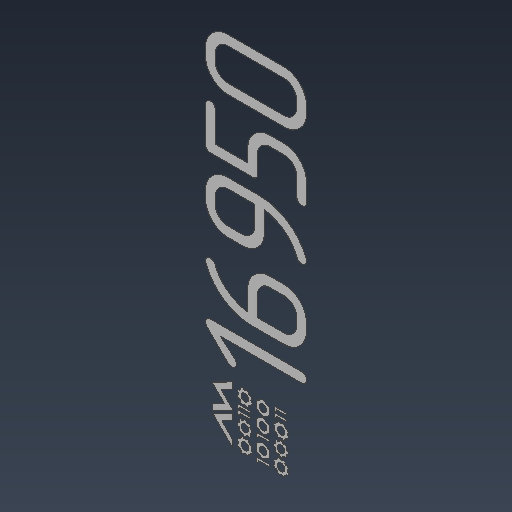
# Autodesk Inventor part: цифры
Saved by Autodesk Inventor 2025 (Build 290162000, 162)
## iProperties
Created: 2025-03-07
Part Number: цифры
Material: Типовые
Document SubType Name: Modeling
Designer: GameHD
Density: 1 g/cm^3
Appearance: По умолчанию
Author: GameHD
Autodesk Inventor part; units mm, degrees
ref_plane "YZ Plane" through (0, 0, 0) normal (1, 0, 0) x (0, 1, 0)
ref_plane "XZ Plane" through (0, 0, 0) normal (0, 1, 0) x (-1, 0, 0)
ref_plane "XY Plane" through (0, 0, 0) normal (0, 0, 1) x (1, 0, 0)
sketch "Эскиз1" plane through (0, 0, 0) normal (0, 0, 1) x (1, 0, 0)
  arc A0 (27.3071, -95.8521) -> (31.3071, -91.8521) centre (27.3071, -91.8521) ccw
  line L0 (31.3071, 96.2479) -> (31.3071, -91.8521)
  arc A1 (31.3071, 96.2479) -> (28.3071, 99.2479) centre (28.3071, 96.2479) ccw
  line L1 (-29.1929, 99.2479) -> (28.3071, 99.2479)
  arc A2 (-29.1929, 99.2479) -> (-32.1929, 96.2479) centre (-29.1929, 96.2479) ccw
  line L2 (-32.1929, -91.8521) -> (-32.1929, 96.2479)
  arc A3 (-32.1929, -91.8521) -> (-28.1929, -95.8521) centre (-28.1929, -91.8521) ccw
  line L3 (-28.1929, -95.8521) -> (27.3071, -95.8521)
  line L4 (-18.208, -66.6682) -> (-12.464, -72.4126)
  line L5 (-12.464, -72.4126) -> (-12.464, -72.9974)
  line L6 (-12.464, -72.9974) -> (-22.3101, -77.9492)
  line L7 (-22.3101, -77.9492) -> (-22.3101, -74.8598)
  line L8 (-22.3101, -74.8598) -> (-16.5747, -71.9754)
  line L9 (-16.5747, -71.9754) -> (-22.3101, -66.2395)
  line L10 (-22.3101, -66.2395) -> (-22.3101, -65.617)
  line L11 (-22.3101, -65.617) -> (-12.464, -60.6652)
  line L12 (-12.464, -60.6652) -> (-12.485, -63.79)
  line L13 (-12.485, -63.79) -> (-18.208, -66.6682)
  line L14 (-5.5283, -89.0998) -> (-5.7626, -88.5746)
  arc A4 (-6.7374, -88.5729) -> (-5.7626, -88.5746) centre (-6.2446, -85.4284) ccw
  line L15 (-6.7374, -88.5729) -> (-6.9459, -89.1173)
  arc A5 (-8.3342, -88.531) -> (-6.9459, -89.1173) centre (-6.8364, -86.9215) ccw
  line L16 (-8.3342, -88.531) -> (-8.1285, -87.9939)
  arc A6 (-8.8166, -87.3034) -> (-8.1285, -87.9939) centre (-6.2446, -85.4284) ccw
  line L17 (-8.8166, -87.3034) -> (-9.349, -87.5409)
  arc A7 (-9.916, -86.1447) -> (-9.349, -87.5409) centre (-7.7189, -86.0657) ccw
  line L18 (-9.916, -86.1447) -> (-9.3907, -85.9104)
  arc A8 (-9.3891, -84.9356) -> (-9.3907, -85.9104) centre (-6.2446, -85.4284) ccw
  line L19 (-9.3891, -84.9356) -> (-9.9335, -84.7271)
  arc A9 (-9.3471, -83.3388) -> (-9.9335, -84.7271) centre (-7.7377, -84.8366) ccw
  line L20 (-9.3471, -83.3388) -> (-8.81, -83.5445)
  arc A10 (-8.1196, -82.8564) -> (-8.81, -83.5445) centre (-6.2446, -85.4284) ccw
  line L21 (-8.1196, -82.8564) -> (-8.3571, -82.324)
  arc A11 (-6.9608, -81.757) -> (-8.3571, -82.324) centre (-6.8819, -83.9541) ccw
  line L22 (-6.9608, -81.757) -> (-6.7265, -82.2822)
  arc A12 (-5.7517, -82.2839) -> (-6.7265, -82.2822) centre (-6.2446, -85.4284) ccw
  line L23 (-5.7517, -82.2839) -> (-5.5432, -81.7395)
  arc A13 (-4.155, -82.3259) -> (-5.5432, -81.7395) centre (-5.6527, -83.9353) ccw
  line L24 (-4.155, -82.3259) -> (-4.3713, -82.8744)
  arc A14 (-3.6832, -83.5648) -> (-4.3713, -82.8744) centre (-6.2552, -85.4398) ccw
  line L25 (-3.6832, -83.5648) -> (-3.1508, -83.3273)
  arc A15 (-2.5838, -84.7236) -> (-3.1508, -83.3273) centre (-4.7809, -84.8025) ccw
  line L26 (-2.5838, -84.7236) -> (-3.109, -84.9579)
  arc A16 (-3.1107, -85.9327) -> (-3.109, -84.9579) centre (-6.2552, -85.4398) ccw
  line L27 (-3.1107, -85.9327) -> (-2.5663, -86.1412)
  arc A17 (-3.142, -87.518) -> (-2.5663, -86.1412) centre (-4.7621, -86.0318) ccw
  line L28 (-3.142, -87.518) -> (-3.6791, -87.3123)
  arc A18 (-4.3696, -88.0004) -> (-3.6791, -87.3123) centre (-6.2446, -85.4284) ccw
  line L29 (-4.3696, -88.0004) -> (-4.132, -88.5328)
  arc A19 (-5.5283, -89.0998) -> (-4.132, -88.5328) centre (-5.6073, -86.9027) ccw
  line L30 (-9.8069, -73.459) -> (-9.8069, -71.4081)
  line L31 (-9.8069, -71.4081) -> (-3.4639, -71.4081)
  line L32 (-3.4639, -71.4081) -> (-3.4639, -72.491)
  line L33 (-3.4639, -72.491) -> (-8.6953, -72.491)
  line L34 (-8.6953, -72.491) -> (-8.6953, -73.459)
  line L35 (-8.6953, -73.459) -> (-9.8069, -73.459)
  line L36 (-0.4429, -89.1671) -> (-0.4429, -87.1162)
  line L37 (-0.4429, -87.1162) -> (5.9001, -87.1162)
  line L38 (5.9001, -87.1162) -> (5.9001, -88.1992)
  line L39 (5.9001, -88.1992) -> (0.6687, -88.1992)
  line L40 (0.6687, -88.1992) -> (0.6687, -89.1671)
  line L41 (0.6687, -89.1671) -> (-0.4429, -89.1671)
  line L42 (8.3427, -65.5184) -> (8.3427, -63.4675)
  line L43 (8.3427, -63.4675) -> (14.6857, -63.4675)
  line L44 (14.6857, -63.4675) -> (14.6857, -64.5504)
  line L45 (14.6857, -64.5504) -> (9.4543, -64.5504)
  line L46 (9.4543, -64.5504) -> (9.4543, -65.5184)
  line L47 (9.4543, -65.5184) -> (8.3427, -65.5184)
  arc A20 (11.322, -88.5729) -> (12.2968, -88.5746) centre (11.8148, -85.4284) ccw
  line L48 (11.322, -88.5729) -> (11.1135, -89.1173)
  arc A21 (9.7252, -88.531) -> (11.1135, -89.1173) centre (11.223, -86.9215) ccw
  line L49 (9.7252, -88.531) -> (9.9309, -87.9939)
  arc A22 (9.2428, -87.3034) -> (9.9309, -87.9939) centre (11.8148, -85.4284) ccw
  line L50 (9.2428, -87.3034) -> (8.7104, -87.5409)
  arc A23 (8.1434, -86.1447) -> (8.7104, -87.5409) centre (10.3405, -86.0657) ccw
  line L51 (8.1434, -86.1447) -> (8.6686, -85.9104)
  arc A24 (8.6703, -84.9356) -> (8.6686, -85.9104) centre (11.8148, -85.4284) ccw
  line L52 (8.6703, -84.9356) -> (8.1259, -84.7271)
  arc A25 (8.7123, -83.3388) -> (8.1259, -84.7271) centre (10.3217, -84.8366) ccw
  line L53 (8.7123, -83.3388) -> (9.2493, -83.5445)
  arc A26 (9.9398, -82.8564) -> (9.2493, -83.5445) centre (11.8148, -85.4284) ccw
  line L54 (9.9398, -82.8564) -> (9.7023, -82.324)
  arc A27 (11.0986, -81.757) -> (9.7023, -82.324) centre (11.1775, -83.9541) ccw
  line L55 (11.0986, -81.757) -> (11.3329, -82.2822)
  arc A28 (12.3077, -82.2839) -> (11.3329, -82.2822) centre (11.8148, -85.4284) ccw
  line L56 (12.3077, -82.2839) -> (12.5162, -81.7395)
  arc A29 (13.9044, -82.3259) -> (12.5162, -81.7395) centre (12.4067, -83.9353) ccw
  line L57 (13.9044, -82.3259) -> (13.6987, -82.8629)
  arc A30 (14.3868, -83.5534) -> (13.6987, -82.8629) centre (11.8148, -85.4284) ccw
  line L58 (14.3868, -83.5534) -> (14.9192, -83.3159)
  arc A31 (15.4862, -84.7122) -> (14.9192, -83.3159) centre (13.2891, -84.7911) ccw
  line L59 (15.4862, -84.7122) -> (14.961, -84.9465)
  arc A32 (14.9593, -85.9213) -> (14.961, -84.9465) centre (11.8148, -85.4284) ccw
  line L60 (14.9593, -85.9213) -> (15.5037, -86.1298)
  arc A33 (14.9174, -87.518) -> (15.5037, -86.1298) centre (13.3079, -86.0203) ccw
  line L61 (14.9174, -87.518) -> (14.3803, -87.3123)
  arc A34 (13.6898, -88.0004) -> (14.3803, -87.3123) centre (11.8148, -85.4284) ccw
  line L62 (13.6898, -88.0004) -> (13.9273, -88.5328)
  arc A35 (12.5311, -89.0998) -> (13.9273, -88.5328) centre (12.4521, -86.9027) ccw
  line L63 (12.5311, -89.0998) -> (12.2968, -88.5746)
  line L64 (8.3427, -62.7161) -> (8.3427, -60.6652)
  line L65 (8.3427, -60.6652) -> (14.6857, -60.6652)
  line L66 (14.6857, -60.6652) -> (14.6857, -61.7481)
  line L67 (14.6857, -61.7481) -> (9.4543, -61.7481)
  line L68 (9.4543, -61.7481) -> (9.4543, -62.7161)
  line L69 (9.4543, -62.7161) -> (8.3427, -62.7161)
  line L70 (-0.4429, -78.55) -> (-0.4429, -76.4991)
  line L71 (-0.4429, -76.4991) -> (5.9001, -76.4991)
  line L72 (5.9001, -76.4991) -> (5.9001, -77.5821)
  line L73 (5.9001, -77.5821) -> (0.6687, -77.5821)
  line L74 (0.6687, -77.5821) -> (0.6687, -78.55)
  line L75 (0.6687, -78.55) -> (-0.4429, -78.55)
  line L76 (-3.4639, -69.8464) -> (-8.6953, -69.8464)
  line L77 (-8.6953, -69.8464) -> (-8.6953, -70.8144)
  line L78 (-8.6953, -70.8144) -> (-9.8069, -70.8144)
  line L79 (-9.8069, -70.8144) -> (-9.8069, -68.7635)
  line L80 (-9.8069, -68.7635) -> (-3.4639, -68.7635)
  line L81 (-3.4639, -68.7635) -> (-3.4639, -69.8464)
  line L82 (-22.3101, -79.2695) -> (-12.464, -74.2847)
  line L83 (-12.464, -74.2847) -> (-12.464, -77.3998)
  line L84 (-12.464, -77.3998) -> (-17.7048, -80.0531)
  line L85 (-17.7048, -80.0531) -> (-12.464, -85.531)
  line L86 (-12.464, -85.531) -> (-12.464, -89.0892)
  line L87 (-12.464, -89.0892) -> (-22.3101, -79.2695)
  arc A36 (-7.8758, -80.1695) -> (-7.029, -80.513) centre (-6.3219, -77.554) ccw
  line L88 (-7.8758, -80.1695) -> (-8.3322, -80.5742)
  arc A37 (-9.3244, -79.5396) -> (-8.3322, -80.5742) centre (-7.1141, -78.4131) ccw
  line L89 (-9.3244, -79.5396) -> (-8.9143, -79.1463)
  arc A38 (-9.2702, -78.3047) -> (-8.9143, -79.1463) centre (-6.3219, -77.554) ccw
  line L90 (-9.2702, -78.3047) -> (-9.8791, -78.2681)
  arc A39 (-9.849, -76.8349) -> (-9.8791, -78.2681) centre (-7.4896, -77.6013) ccw
  line L91 (-9.849, -76.8349) -> (-9.2809, -76.8468)
  arc A40 (-8.9375, -76.0001) -> (-9.2809, -76.8468) centre (-6.3219, -77.554) ccw
  line L92 (-8.9375, -76.0001) -> (-9.3422, -75.5437)
  arc A41 (-8.3075, -74.5515) -> (-9.3422, -75.5437) centre (-7.1811, -76.7617) ccw
  line L93 (-8.3075, -74.5515) -> (-7.9143, -74.9616)
  arc A42 (-7.0727, -74.6057) -> (-7.9143, -74.9616) centre (-6.3219, -77.554) ccw
  line L94 (-7.0727, -74.6057) -> (-7.0361, -73.9968)
  arc A43 (-5.6029, -74.0268) -> (-7.0361, -73.9968) centre (-6.3693, -76.3863) ccw
  line L95 (-5.6029, -74.0268) -> (-5.6148, -74.5949)
  arc A44 (-4.7681, -74.9384) -> (-5.6148, -74.5949) centre (-6.3219, -77.554) ccw
  line L96 (-4.7681, -74.9384) -> (-4.3116, -74.5337)
  arc A45 (-3.3195, -75.5683) -> (-4.3116, -74.5337) centre (-5.5297, -76.6948) ccw
  line L97 (-3.3195, -75.5683) -> (-3.7296, -75.9616)
  arc A46 (-3.3737, -76.8032) -> (-3.7296, -75.9616) centre (-6.3219, -77.554) ccw
  line L98 (-3.3737, -76.8032) -> (-2.7648, -76.8398)
  arc A47 (-2.7948, -78.273) -> (-2.7648, -76.8398) centre (-5.1542, -77.5066) ccw
  line L99 (-2.7948, -78.273) -> (-3.3629, -78.2611)
  arc A48 (-3.7063, -79.1078) -> (-3.3629, -78.2611) centre (-6.3219, -77.554) ccw
  line L100 (-3.7063, -79.1078) -> (-3.3016, -79.5642)
  arc A49 (-4.3363, -80.5564) -> (-3.3016, -79.5642) centre (-5.4628, -78.3462) ccw
  line L101 (-4.3363, -80.5564) -> (-4.7296, -80.1463)
  arc A50 (-5.5712, -80.5022) -> (-4.7296, -80.1463) centre (-6.3219, -77.554) ccw
  line L102 (-5.5712, -80.5022) -> (-5.6078, -81.1111)
  arc A51 (-7.0409, -81.0811) -> (-5.6078, -81.1111) centre (-6.2746, -78.7216) ccw
  line L103 (-7.0409, -81.0811) -> (-7.029, -80.513)
  line L104 (5.9001, -80.9599) -> (5.9001, -84.6242)
  line L105 (5.9001, -84.6242) -> (2.6904, -86.4378)
  line L106 (2.6904, -86.4378) -> (-0.4429, -84.6242)
  line L107 (-0.4429, -84.6242) -> (-0.4429, -80.9599)
  line L108 (-0.4429, -80.9599) -> (2.7668, -79.1463)
  line L109 (2.7668, -79.1463) -> (5.9001, -80.9599)
  line L110 (2.7668, -60.7467) -> (5.9001, -62.5603)
  line L111 (5.9001, -62.5603) -> (5.9001, -66.2246)
  line L112 (5.9001, -66.2246) -> (2.6904, -68.0382)
  line L113 (2.6904, -68.0382) -> (-0.4429, -66.2246)
  line L114 (-0.4429, -66.2246) -> (-0.4429, -62.5603)
  line L115 (-0.4429, -62.5603) -> (2.7668, -60.7467)
  arc A52 (12.4882, -80.5022) -> (13.3298, -80.1463) centre (11.7375, -77.554) ccw
  line L116 (12.4882, -80.5022) -> (12.4516, -81.1111)
  arc A53 (11.0184, -81.0811) -> (12.4516, -81.1111) centre (11.7848, -78.7216) ccw
  line L117 (11.0184, -81.0811) -> (11.0303, -80.513)
  arc A54 (10.1836, -80.1695) -> (11.0303, -80.513) centre (11.7375, -77.554) ccw
  line L118 (10.1836, -80.1695) -> (9.7272, -80.5742)
  arc A55 (8.735, -79.5396) -> (9.7272, -80.5742) centre (10.9453, -78.4131) ccw
  line L119 (8.735, -79.5396) -> (9.1451, -79.1463)
  arc A56 (8.7892, -78.3047) -> (9.1451, -79.1463) centre (11.7375, -77.554) ccw
  line L120 (8.7892, -78.3047) -> (8.1803, -78.2681)
  arc A57 (8.2104, -76.8349) -> (8.1803, -78.2681) centre (10.5698, -77.6013) ccw
  line L121 (8.2104, -76.8349) -> (8.7784, -76.8468)
  arc A58 (9.1219, -76.0001) -> (8.7784, -76.8468) centre (11.7375, -77.554) ccw
  line L122 (9.1219, -76.0001) -> (8.7172, -75.5437)
  arc A59 (9.7518, -74.5515) -> (8.7172, -75.5437) centre (10.8783, -76.7617) ccw
  line L123 (9.7518, -74.5515) -> (10.1451, -74.9616)
  arc A60 (10.9867, -74.6057) -> (10.1451, -74.9616) centre (11.7375, -77.554) ccw
  line L124 (10.9867, -74.6057) -> (11.0233, -73.9968)
  arc A61 (12.4565, -74.0268) -> (11.0233, -73.9968) centre (11.6901, -76.3863) ccw
  line L125 (12.4565, -74.0268) -> (12.4446, -74.5949)
  arc A62 (13.2913, -74.9384) -> (12.4446, -74.5949) centre (11.7375, -77.554) ccw
  line L126 (13.2913, -74.9384) -> (13.7478, -74.5337)
  arc A63 (14.7399, -75.5683) -> (13.7478, -74.5337) centre (12.5297, -76.6948) ccw
  line L127 (14.7399, -75.5683) -> (14.3298, -75.9616)
  arc A64 (14.6857, -76.8032) -> (14.3298, -75.9616) centre (11.7375, -77.554) ccw
  line L128 (14.6857, -76.8032) -> (15.2946, -76.8398)
  arc A65 (15.2646, -78.273) -> (15.2946, -76.8398) centre (12.9052, -77.5066) ccw
  line L129 (15.2646, -78.273) -> (14.6965, -78.2611)
  arc A66 (14.353, -79.1078) -> (14.6965, -78.2611) centre (11.7375, -77.554) ccw
  line L130 (14.353, -79.1078) -> (14.7577, -79.5642)
  arc A67 (13.7231, -80.5564) -> (14.7577, -79.5642) centre (12.5966, -78.3462) ccw
  line L131 (13.7231, -80.5564) -> (13.3298, -80.1463)
  arc A68 (12.5311, -73.312) -> (13.9273, -72.745) centre (12.4521, -71.1149) ccw
  line L132 (12.5311, -73.312) -> (12.2968, -72.7868)
  arc A69 (11.322, -72.7851) -> (12.2968, -72.7868) centre (11.8148, -69.6406) ccw
  line L133 (11.322, -72.7851) -> (11.1135, -73.3295)
  arc A70 (9.7252, -72.7431) -> (11.1135, -73.3295) centre (11.223, -71.1337) ccw
  line L134 (9.7252, -72.7431) -> (9.9309, -72.2061)
  arc A71 (9.2428, -71.5156) -> (9.9309, -72.2061) centre (11.8148, -69.6406) ccw
  line L135 (9.2428, -71.5156) -> (8.7104, -71.7531)
  arc A72 (8.1434, -70.3569) -> (8.7104, -71.7531) centre (10.3405, -70.2779) ccw
  line L136 (8.1434, -70.3569) -> (8.6686, -70.1226)
  arc A73 (8.6703, -69.1478) -> (8.6686, -70.1226) centre (11.8148, -69.6406) ccw
  line L137 (8.6703, -69.1478) -> (8.1259, -68.9393)
  arc A74 (8.7123, -67.551) -> (8.1259, -68.9393) centre (10.3217, -69.0488) ccw
  line L138 (8.7123, -67.551) -> (9.2493, -67.7567)
  arc A75 (9.9398, -67.0686) -> (9.2493, -67.7567) centre (11.8148, -69.6406) ccw
  line L139 (9.9398, -67.0686) -> (9.7023, -66.5362)
  arc A76 (11.0986, -65.9692) -> (9.7023, -66.5362) centre (11.1775, -68.1663) ccw
  line L140 (11.0986, -65.9692) -> (11.3329, -66.4944)
  arc A77 (12.3077, -66.4961) -> (11.3329, -66.4944) centre (11.8148, -69.6406) ccw
  line L141 (12.3077, -66.4961) -> (12.5162, -65.9517)
  arc A78 (13.9044, -66.5381) -> (12.5162, -65.9517) centre (12.4067, -68.1475) ccw
  line L142 (13.9044, -66.5381) -> (13.6987, -67.0751)
  arc A79 (14.3868, -67.7656) -> (13.6987, -67.0751) centre (11.8148, -69.6406) ccw
  line L143 (14.3868, -67.7656) -> (14.9192, -67.5281)
  arc A80 (15.4862, -68.9243) -> (14.9192, -67.5281) centre (13.2891, -69.0033) ccw
  line L144 (15.4862, -68.9243) -> (14.961, -69.1587)
  arc A81 (14.9593, -70.1334) -> (14.961, -69.1587) centre (11.8148, -69.6406) ccw
  line L145 (14.9593, -70.1334) -> (15.5037, -70.342)
  arc A82 (14.9174, -71.7302) -> (15.5037, -70.342) centre (13.3079, -70.2325) ccw
  line L146 (14.9174, -71.7302) -> (14.3803, -71.5245)
  arc A83 (13.6898, -72.2126) -> (14.3803, -71.5245) centre (11.8148, -69.6406) ccw
  line L147 (13.6898, -72.2126) -> (13.9273, -72.745)
  line L148 (5.9001, -70.2994) -> (5.9001, -73.9636)
  line L149 (5.9001, -73.9636) -> (2.6904, -75.7772)
  line L150 (2.6904, -75.7772) -> (-0.4429, -73.9636)
  line L151 (-0.4429, -73.9636) -> (-0.4429, -70.2994)
  line L152 (-0.4429, -70.2994) -> (2.7668, -68.4857)
  line L153 (2.7668, -68.4857) -> (5.9001, -70.2994)
  line L154 (-5.6057, -68.021) -> (-5.84, -67.4958)
  arc A84 (-6.8148, -67.4941) -> (-5.84, -67.4958) centre (-6.3219, -64.3496) ccw
  line L155 (-6.8148, -67.4941) -> (-7.0233, -68.0385)
  arc A85 (-8.4115, -67.4521) -> (-7.0233, -68.0385) centre (-6.9138, -65.8427) ccw
  line L156 (-8.4115, -67.4521) -> (-8.2058, -66.9151)
  arc A86 (-8.8939, -66.2246) -> (-8.2058, -66.9151) centre (-6.3219, -64.3496) ccw
  line L157 (-8.8939, -66.2246) -> (-9.4263, -66.4621)
  arc A87 (-9.9933, -65.0658) -> (-9.4263, -66.4621) centre (-7.7962, -64.9869) ccw
  line L158 (-9.9933, -65.0658) -> (-9.4681, -64.8315)
  arc A88 (-9.4664, -63.8567) -> (-9.4681, -64.8315) centre (-6.3219, -64.3496) ccw
  line L159 (-9.4664, -63.8567) -> (-10.0108, -63.6482)
  arc A89 (-9.4245, -62.26) -> (-10.0108, -63.6482) centre (-7.815, -63.7577) ccw
  line L160 (-9.4245, -62.26) -> (-8.8874, -62.4657)
  arc A90 (-8.1969, -61.7776) -> (-8.8874, -62.4657) centre (-6.3219, -64.3496) ccw
  line L161 (-8.1969, -61.7776) -> (-8.4344, -61.2452)
  arc A91 (-7.0382, -60.6782) -> (-8.4344, -61.2452) centre (-6.9592, -62.8753) ccw
  line L162 (-7.0382, -60.6782) -> (-6.8039, -61.2034)
  arc A92 (-5.8291, -61.2051) -> (-6.8039, -61.2034) centre (-6.3219, -64.3496) ccw
  line L163 (-5.8291, -61.2051) -> (-5.6206, -60.6607)
  arc A93 (-4.2323, -61.247) -> (-5.6206, -60.6607) centre (-5.7301, -62.8565) ccw
  line L164 (-4.2323, -61.247) -> (-4.438, -61.7841)
  arc A94 (-3.7499, -62.4746) -> (-4.438, -61.7841) centre (-6.3219, -64.3496) ccw
  line L165 (-3.7499, -62.4746) -> (-3.2175, -62.2371)
  arc A95 (-2.6505, -63.6333) -> (-3.2175, -62.2371) centre (-4.8476, -63.7123) ccw
  line L166 (-2.6505, -63.6333) -> (-3.1757, -63.8676)
  arc A96 (-3.1774, -64.8424) -> (-3.1757, -63.8676) centre (-6.3219, -64.3496) ccw
  line L167 (-3.1774, -64.8424) -> (-2.633, -65.0509)
  arc A97 (-3.2194, -66.4392) -> (-2.633, -65.0509) centre (-4.8288, -64.9414) ccw
  line L168 (-3.2194, -66.4392) -> (-3.7565, -66.2335)
  arc A98 (-4.4469, -66.9216) -> (-3.7565, -66.2335) centre (-6.3219, -64.3496) ccw
  line L169 (-4.4469, -66.9216) -> (-4.2094, -67.454)
  arc A99 (-5.6057, -68.021) -> (-4.2094, -67.454) centre (-5.6846, -65.8239) ccw
  spline S0 degree 3 poles (23.895, -39.5819) (23.4468, -39.1337) (22.8405, -38.9095) (22.0761, -38.9095) knots 0 0 0 0 1 1 1 1
  spline S1 degree 3 poles (24.5598, -41.4041) (24.5598, -40.7065) (24.3382, -40.099) (23.895, -39.5819) knots 0 0 0 0 1 1 1 1
  spline S2 degree 3 poles (24.0603, -42.9868) (24.3933, -42.2651) (24.5598, -41.7376) (24.5598, -41.4041) knots 0 0 0 0 1 1 1 1
  spline S3 degree 3 poles (22.0761, -43.888) (22.9182, -43.888) (23.5796, -43.5876) (24.0603, -42.9868) knots 0 0 0 0 1 1 1 1
  line L170 (-18.5493, -43.888) -> (22.0761, -43.888)
  line L171 (-11.2202, -50.1309) -> (-18.5493, -43.888)
  spline S4 degree 3 poles (-10.4888, -51.8435) (-10.4888, -51.189) (-10.7326, -50.6182) (-11.2202, -50.1309) knots 0 0 0 0 1 1 1 1
  spline S5 degree 3 poles (-11.2204, -53.6302) (-10.7327, -53.1429) (-10.4888, -52.5473) (-10.4888, -51.8435) knots 0 0 0 0 1 1 1 1
  spline S6 degree 3 poles (-13.0081, -54.3611) (-12.3041, -54.3611) (-11.7082, -54.1175) (-11.2204, -53.6302) knots 0 0 0 0 1 1 1 1
  spline S7 degree 3 poles (-14.6619, -53.6822) (-13.8767, -54.1348) (-13.3255, -54.3611) (-13.0081, -54.3611) knots 0 0 0 0 1 1 1 1
  line L172 (-25.2323, -43.1548) -> (-14.6619, -53.6822)
  spline S8 degree 3 poles (-25.9401, -41.4383) (-25.9401, -42.1111) (-25.7041, -42.6833) (-25.2323, -43.1548) knots 0 0 0 0 1 1 1 1
  spline S9 degree 3 poles (-25.2643, -39.685) (-25.7148, -40.2019) (-25.9401, -40.7864) (-25.9401, -41.4383) knots 0 0 0 0 1 1 1 1
  spline S10 degree 3 poles (-23.4913, -38.9095) (-24.2228, -38.9095) (-24.8138, -39.168) (-25.2643, -39.685) knots 0 0 0 0 1 1 1 1
  line L173 (22.0761, -38.9095) -> (-23.4913, -38.9095)
  spline S11 degree 3 poles (21.2422, 52.1802) (19.0322, 54.3783) (16.3891, 55.4774) (13.3129, 55.4774) knots -0.892114 -0.892114 -0.892114 -0.892114 0 0 0 0
  spline S12 degree 3 poles (24.5571, 44.2544) (24.5571, 47.3402) (23.4522, 49.9822) (21.2422, 52.1802) knots -0.892943 -0.892943 -0.892943 -0.892943 0 0 0 0
  line L174 (24.5571, 35.4559) -> (24.5571, 44.2544)
  spline S13 degree 3 poles (23.8646, 33.6372) (24.3263, 34.0989) (24.5571, 34.7051) (24.5571, 35.4559) knots 0 0 0 0 1 1 1 1
  spline S14 degree 3 poles (22.0733, 32.972) (22.7217, 32.972) (23.3188, 33.1938) (23.8646, 33.6372) knots 0 0 0 0 1 1 1 1
  spline S15 degree 3 poles (20.5334, 33.5772) (21.1628, 33.1738) (21.6761, 32.972) (22.0733, 32.972) knots 0 0 0 0 1 1 1 1
  spline S16 degree 3 poles (19.5894, 35.4559) (19.5894, 34.6069) (19.9041, 33.9807) (20.5334, 33.5772) knots 0 0 0 0 1 1 1 1
  line L175 (19.5894, 44.2544) -> (19.5894, 35.4559)
  spline S17 degree 3 poles (17.7684, 48.6771) (18.9824, 47.4627) (19.5894, 45.9884) (19.5894, 44.2544) knots 0 0 0 0 1 1 1 1
  spline S18 degree 3 poles (13.3125, 50.4989) (15.0691, 50.4989) (16.5544, 49.8916) (17.7684, 48.6771) knots -0.500222 -0.500222 -0.500222 -0.500222 0 0 0 0
  line L176 (6.3045, 50.4989) -> (13.3125, 50.4989)
  spline S19 degree 3 poles (1.8893, 48.6714) (3.107, 49.8897) (4.5788, 50.4989) (6.3045, 50.4989) knots 0 0 0 0 1 1 1 1
  spline S20 degree 3 poles (0.0626, 44.2544) (0.0626, 45.9808) (0.6715, 47.4531) (1.8893, 48.6714) knots 0 0 0 0 1 1 1 1
  line L177 (0.0626, 35.4559) -> (0.0626, 44.2544)
  spline S21 degree 3 poles (-2.4211, 32.972) (-0.7653, 32.972) (0.0626, 33.8) (0.0626, 35.4559) knots 0 0 0 0 1 1 1 1
  line L178 (-23.486, 32.972) -> (-2.4211, 32.972)
  spline S22 degree 3 poles (-25.9696, 35.4559) (-25.9696, 33.8) (-25.1417, 32.972) (-23.486, 32.972) knots 0 0 0 0 1 1 1 1
  line L179 (-25.9696, 52.9828) -> (-25.9696, 35.4559)
  spline S23 degree 3 poles (-25.1902, 54.6979) (-25.7098, 54.1782) (-25.9696, 53.6065) (-25.9696, 52.9828) knots 0 0 0 0 1 1 1 1
  spline S24 degree 3 poles (-23.4858, 55.4774) (-24.1024, 55.4774) (-24.6705, 55.2175) (-25.1902, 54.6979) knots 0 0 0 0 1 1 1 1
  spline S25 degree 3 poles (-21.8011, 54.8279) (-22.334, 55.2609) (-22.8955, 55.4774) (-23.4858, 55.4774) knots 0 0 0 0 1 1 1 1
  spline S26 degree 3 poles (-21.0019, 52.9828) (-21.0019, 53.7799) (-21.2683, 54.395) (-21.8011, 54.8279) knots 0 0 0 0 1 1 1 1
  line L180 (-21.0019, 37.9505) -> (-21.0019, 52.9828)
  line L181 (-4.9052, 37.9505) -> (-21.0019, 37.9505)
  line L182 (-4.9052, 44.2544) -> (-4.9052, 37.9505)
  spline S27 degree 3 poles (-1.6027, 52.1739) (-3.8043, 49.9717) (-4.9052, 47.3318) (-4.9052, 44.2544) knots -0.891608 -0.891608 -0.891608 -0.891608 0 0 0 0
  spline S28 degree 3 poles (6.3041, 55.4774) (3.2346, 55.4774) (0.599, 54.3762) (-1.6027, 52.1739) knots -0.890428 -0.890428 -0.890428 -0.890428 0 0 0 0
  line L183 (13.3129, 55.4774) -> (6.3041, 55.4774)
  spline S29 degree 3 poles (24.5571, 77.293) (24.5571, 80.4253) (23.4521, 83.0903) (21.242, 85.2881) knots -0.899625 -0.899625 -0.899625 -0.899625 0 0 0 0
  line L184 (24.5571, 73.788) -> (24.5571, 77.293)
  spline S30 degree 3 poles (21.3036, 66.0015) (23.4726, 68.3078) (24.5571, 70.9034) (24.5571, 73.788) knots -0.873729 -0.873729 -0.873729 -0.873729 0 0 0 0
  spline S31 degree 3 poles (13.3122, 62.5419) (16.4708, 62.5419) (19.1346, 63.6951) (21.3036, 66.0015) knots -0.903236 -0.903236 -0.903236 -0.903236 0 0 0 0
  line L185 (-14.7247, 62.5419) -> (13.3122, 62.5419)
  spline S32 degree 3 poles (-22.6008, 65.7988) (-20.3549, 63.6275) (-17.7295, 62.5419) (-14.7247, 62.5419) knots -0.884105 -0.884105 -0.884105 -0.884105 0 0 0 0
  spline S33 degree 3 poles (-25.9696, 73.788) (-25.9696, 70.6331) (-24.8467, 67.97) (-22.6008, 65.7988) knots -0.89849 -0.89849 -0.89849 -0.89849 0 0 0 0
  line L186 (-25.9696, 77.293) -> (-25.9696, 73.788)
  spline S34 degree 3 poles (-22.6806, 85.2391) (-24.8733, 83.0086) (-25.9696, 80.3599) (-25.9696, 77.293) knots -0.892879 -0.892879 -0.892879 -0.892879 0 0 0 0
  spline S35 degree 3 poles (-14.7247, 88.5848) (-17.8359, 88.5848) (-20.4879, 87.4696) (-22.6806, 85.2391) knots -0.897588 -0.897588 -0.897588 -0.897588 0 0 0 0
  line L187 (13.3122, 88.5848) -> (-14.7247, 88.5848)
  spline S36 degree 3 poles (21.242, 85.2881) (19.032, 87.4859) (16.3887, 88.5848) (13.3122, 88.5848) knots -0.892138 -0.892138 -0.892138 -0.892138 0 0 0 0
  spline S37 degree 3 poles (24.4187, 11.0665) (22.4321, 16.1074) (19.1741, 20.0378) (14.6445, 22.8578) knots -1.570967 -1.570967 -1.570967 -1.570967 0 0 0 0
  line L188 (24.5894, 10.1693) -> (24.4187, 11.0665)
  spline S38 degree 3 poles (23.8938, 8.4145) (24.3575, 9.1565) (24.5894, 9.7415) (24.5894, 10.1693) knots 0 0 0 0 1 1 1 1
  spline S39 degree 3 poles (22.0356, 7.7233) (22.7074, 7.7233) (23.3268, 7.9537) (23.8938, 8.4145) knots 0 0 0 0 1 1 1 1
  spline S40 degree 3 poles (20.7028, 8.0368) (21.1186, 7.8278) (21.5628, 7.7233) (22.0356, 7.7233) knots 0 0 0 0 1 1 1 1
  spline S41 degree 3 poles (19.932, 8.8508) (20.0301, 8.5171) (20.287, 8.2458) (20.7028, 8.0368) knots 0 0 0 0 1 1 1 1
  spline S42 degree 3 poles (18.5308, 11.926) (19.0696, 10.9831) (19.5367, 9.958) (19.932, 8.8508) knots 0 0 0 0 1 1 1 1
  line L189 (17.523, 13.5297) -> (18.5308, 11.926)
  line L190 (17.3233, 13.8199) -> (17.523, 13.5297)
  line L191 (16.5738, 14.7241) -> (17.3233, 13.8199)
  spline S43 degree 3 poles (12.0338, 18.6655) (14.0041, 17.36) (15.5174, 16.0462) (16.5738, 14.7241) knots -0.599768 -0.599768 -0.599768 -0.599768 0 0 0 0
  spline S44 degree 3 poles (7.4209, 20.8204) (9.0924, 20.2031) (10.63, 19.4848) (12.0338, 18.6655) knots -0.509776 -0.509776 -0.509776 -0.509776 0 0 0 0
  spline S45 degree 3 poles (3.5249, 21.7463) (4.4508, 21.7463) (5.7494, 21.4376) (7.4209, 20.8204) knots 0 0 0 0 1 1 1 1
  line L192 (3.5249, 11.9964) -> (3.5249, 21.7463)
  spline S46 degree 3 poles (0.2712, 3.98) (2.4404, 6.1573) (3.5249, 8.8294) (3.5249, 11.9964) knots -0.898749 -0.898749 -0.898749 -0.898749 0 0 0 0
  spline S47 degree 3 poles (-7.7183, 0.714) (-4.5611, 0.714) (-1.8979, 1.8027) (0.2712, 3.98) knots -0.897028 -0.897028 -0.897028 -0.897028 0 0 0 0
  line L193 (-14.7264, 0.714) -> (-7.7183, 0.714)
  spline S48 degree 3 poles (-22.5957, 3.986) (-20.3465, 1.8047) (-17.7234, 0.714) (-14.7264, 0.714) knots -0.88416 -0.88416 -0.88416 -0.88416 0 0 0 0
  spline S49 degree 3 poles (-25.9696, 11.9914) (-25.9696, 8.8358) (-24.845, 6.1674) (-22.5957, 3.986) knots -0.900117 -0.900117 -0.900117 -0.900117 0 0 0 0
  line L194 (-25.9696, 15.5069) -> (-25.9696, 11.9914)
  spline S50 degree 3 poles (-22.8858, 23.1337) (-24.9417, 21.125) (-25.9696, 18.5827) (-25.9696, 15.5069) knots -0.851106 -0.851106 -0.851106 -0.851106 0 0 0 0
  spline S51 degree 3 poles (-19.0614, 25.965) (-20.4187, 25.4102) (-21.6935, 24.4665) (-22.8858, 23.1337) knots 0 0 0 0 1 1 1 1
  line L195 (-17.057, 26.5341) -> (-19.0614, 25.965)
  line L196 (-15.8405, 26.7247) -> (-17.057, 26.5341)
  line L197 (0.8693, 26.7247) -> (-15.8405, 26.7247)
  spline S52 degree 3 poles (14.6445, 22.8578) (10.4538, 25.4358) (5.8621, 26.7247) (0.8693, 26.7247) knots -1.458138 -1.458138 -1.458138 -1.458138 0 0 0 0
  spline S53 degree 3 poles (-25.8205, -15.9072) (-23.8351, -20.9432) (-20.5769, -24.8711) (-16.0456, -27.6911) knots -1.570437 -1.570437 -1.570437 -1.570437 0 0 0 0
  line L198 (-26.0019, -14.9538) -> (-25.8205, -15.9072)
  spline S54 degree 3 poles (-25.1997, -13.2245) (-25.7345, -13.6756) (-26.0019, -14.252) (-26.0019, -14.9538) knots 0 0 0 0 1 1 1 1
  spline S55 degree 3 poles (-23.4481, -12.5479) (-24.0811, -12.5479) (-24.665, -12.7734) (-25.1997, -13.2245) knots 0 0 0 0 1 1 1 1
  spline S56 degree 3 poles (-22.2181, -12.8822) (-22.5763, -12.6593) (-22.9863, -12.5479) (-23.4481, -12.5479) knots 0 0 0 0 1 1 1 1
  spline S57 degree 3 poles (-21.1442, -14.1473) (-21.5019, -13.5268) (-21.8598, -13.1051) (-22.2181, -12.8822) knots 0 0 0 0 1 1 1 1
  line L199 (-20.8855, -14.8533) -> (-21.1442, -14.1473)
  line L200 (-20.5357, -15.6268) -> (-20.8855, -14.8533)
  line L201 (-19.8894, -16.8667) -> (-20.5357, -15.6268)
  spline S58 degree 3 poles (-18.1656, -19.3375) (-18.7504, -18.6519) (-19.3249, -17.8283) (-19.8894, -16.8667) knots 0 0 0 0 1 1 1 1
  spline S59 degree 3 poles (-13.3618, -23.5473) (-15.3997, -22.1978) (-17.0009, -20.7945) (-18.1656, -19.3375) knots -0.639025 -0.639025 -0.639025 -0.639025 0 0 0 0
  spline S60 degree 3 poles (-8.8804, -25.6477) (-10.5604, -25.0359) (-12.0542, -24.3357) (-13.3618, -23.5473) knots 0 0 0 0 1 1 1 1
  spline S61 degree 3 poles (-4.9374, -26.5655) (-5.886, -26.5655) (-7.2003, -26.2595) (-8.8804, -25.6477) knots 0 0 0 0 1 1 1 1
  line L202 (-4.9374, -16.8264) -> (-4.9374, -26.5655)
  spline S62 degree 3 poles (-1.6707, -8.8122) (-3.8485, -10.9982) (-4.9374, -13.6696) (-4.9374, -16.8264) knots -0.899077 -0.899077 -0.899077 -0.899077 0 0 0 0
  spline S63 degree 3 poles (6.3058, -5.5333) (3.1659, -5.5333) (0.5071, -6.6262) (-1.6707, -8.8122) knots -0.896316 -0.896316 -0.896316 -0.896316 0 0 0 0
  line L203 (13.3139, -5.5333) -> (6.3058, -5.5333)
  spline S64 degree 3 poles (21.2782, -8.8134) (19.0923, -6.6266) (16.4375, -5.5333) (13.3139, -5.5333) knots -0.895041 -0.895041 -0.895041 -0.895041 0 0 0 0
  spline S65 degree 3 poles (24.5571, -16.7913) (24.5571, -13.6595) (23.4642, -11.0002) (21.2782, -8.8134) knots -0.89627 -0.89627 -0.89627 -0.89627 0 0 0 0
  line L204 (24.5571, -20.2967) -> (24.5571, -16.7913)
  spline S66 degree 3 poles (21.3038, -28.084) (23.4727, -25.7774) (24.5571, -23.1816) (24.5571, -20.2967) knots -0.873797 -0.873797 -0.873797 -0.873797 0 0 0 0
  spline S67 degree 3 poles (13.3127, -31.544) (16.4712, -31.544) (19.1349, -30.3906) (21.3038, -28.084) knots -0.903222 -0.903222 -0.903222 -0.903222 0 0 0 0
  line L205 (-2.2819, -31.544) -> (13.3127, -31.544)
  spline S68 degree 3 poles (-16.0456, -27.6911) (-11.8691, -30.2597) (-7.2812, -31.544) (-2.2819, -31.544) knots -1.456596 -1.456596 -1.456596 -1.456596 0 0 0 0
  circle A100 centre (2.7668, -72.233) radius 1.8803
  circle A101 centre (2.7668, -82.826) radius 1.8775
  circle A102 centre (2.6904, -64.3925) radius 1.8471
  circle A103 centre (-6.2446, -85.4284) radius 1.875
  circle A104 centre (-6.3219, -77.554) radius 1.875
  circle A105 centre (-6.3219, -64.3496) radius 1.875
  circle A106 centre (11.8148, -69.6406) radius 1.875
  circle A107 centre (11.7375, -77.554) radius 1.875
  circle A108 centre (11.8148, -85.4284) radius 1.875
  spline S69 degree 3 poles (17.7273, -24.6712) (16.4858, -25.934) (15.0145, -26.5655) (13.3134, -26.5655) knots 0 0 0 0 1 1 1 1
  spline S70 degree 3 poles (19.5894, -20.2967) (19.5894, -21.9501) (18.9687, -23.4083) (17.7273, -24.6712) knots 0 0 0 0 1 1 1 1
  line L206 (19.5894, -16.7913) -> (19.5894, -20.2967)
  spline S71 degree 3 poles (17.7686, -12.3334) (18.9825, -13.5478) (19.5894, -15.0338) (19.5894, -16.7913) knots -0.500337 -0.500337 -0.500337 -0.500337 0 0 0 0
  spline S72 degree 3 poles (13.3134, -10.5117) (15.0696, -10.5117) (16.5547, -11.119) (17.7686, -12.3334) knots -0.500155 -0.500155 -0.500155 -0.500155 0 0 0 0
  line L207 (6.3063, -10.5117) -> (13.3134, -10.5117)
  spline S73 degree 3 poles (1.8667, -12.3178) (3.091, -11.1137) (4.5709, -10.5117) (6.3063, -10.5117) knots 0 0 0 0 1 1 1 1
  spline S74 degree 3 poles (0.0303, -16.7913) (0.0303, -15.013) (0.6424, -13.5218) (1.8667, -12.3178) knots -0.502852 -0.502852 -0.502852 -0.502852 0 0 0 0
  line L208 (0.0303, -26.5655) -> (0.0303, -16.7913)
  line L209 (13.3134, -26.5655) -> (0.0303, -26.5655)
  spline S75 degree 3 poles (-19.1655, 19.9402) (-17.9412, 21.1442) (-16.4613, 21.7463) (-14.7259, 21.7463) knots 0 0 0 0 1 1 1 1
  spline S76 degree 3 poles (-21.0019, 15.4667) (-21.0019, 17.245) (-20.3898, 18.7362) (-19.1655, 19.9402) knots -0.502852 -0.502852 -0.502852 -0.502852 0 0 0 0
  line L210 (-21.0019, 11.9613) -> (-21.0019, 15.4667)
  spline S77 degree 3 poles (-19.1827, 7.5126) (-20.3955, 8.726) (-21.0019, 10.2089) (-21.0019, 11.9613) knots 0 0 0 0 1 1 1 1
  spline S78 degree 3 poles (-14.7259, 5.6925) (-16.4843, 5.6925) (-17.9699, 6.2992) (-19.1827, 7.5126) knots -0.500242 -0.500242 -0.500242 -0.500242 0 0 0 0
  line L211 (-7.7188, 5.6925) -> (-14.7259, 5.6925)
  spline S79 degree 3 poles (-3.305, 7.5868) (-4.5464, 6.324) (-6.0177, 5.6925) (-7.7188, 5.6925) knots 0 0 0 0 1 1 1 1
  spline S80 degree 3 poles (-1.4428, 11.9613) (-1.4428, 10.3079) (-2.0635, 8.8497) (-3.305, 7.5868) knots 0 0 0 0 1 1 1 1
  line L212 (-1.4428, 21.7463) -> (-1.4428, 11.9613)
  line L213 (-14.7259, 21.7463) -> (-1.4428, 21.7463)
  spline S81 degree 3 poles (-19.1399, 81.7441) (-17.8986, 82.9856) (-16.4267, 83.6063) (-14.7242, 83.6063) knots 0 0 0 0 1 1 1 1
  spline S82 degree 3 poles (-21.0019, 77.2928) (-21.0019, 79.0189) (-20.3813, 80.5026) (-19.1399, 81.7441) knots -0.501356 -0.501356 -0.501356 -0.501356 0 0 0 0
  line L214 (-21.0019, 73.788) -> (-21.0019, 77.2928)
  spline S83 degree 3 poles (-19.1647, 69.3577) (-20.3895, 70.5826) (-21.0019, 72.0594) (-21.0019, 73.788) knots 0 0 0 0 1 1 1 1
  spline S84 degree 3 poles (-14.7242, 67.5204) (-16.4598, 67.5204) (-17.9399, 68.1328) (-19.1647, 69.3577) knots 0 0 0 0 1 1 1 1
  line L215 (13.3117, 67.5204) -> (-14.7242, 67.5204)
  spline S85 degree 3 poles (17.7268, 69.4145) (16.485, 68.1517) (15.0133, 67.5204) (13.3117, 67.5204) knots 0 0 0 0 1 1 1 1
  spline S86 degree 3 poles (19.5894, 73.788) (19.5894, 72.1351) (18.9685, 70.6773) (17.7268, 69.4145) knots 0 0 0 0 1 1 1 1
  line L216 (19.5894, 77.2928) -> (19.5894, 73.788)
  spline S87 degree 3 poles (17.7977, 81.7203) (18.9922, 80.4629) (19.5894, 78.9871) (19.5894, 77.2928) knots 0 0 0 0 1 1 1 1
  spline S88 degree 3 poles (13.3117, 83.6063) (15.1079, 83.6063) (16.6033, 82.9776) (17.7977, 81.7203) knots -0.504657 -0.504657 -0.504657 -0.504657 0 0 0 0
  line L217 (-14.7242, 83.6063) -> (13.3117, 83.6063)
  point P0 (0, 0)
  point P1 (-0.4429, 16.6979)
  constraints: 436 end point, 200 point on circle, 109 centre point, 267 other
extrude "Выдавливание1" add sketch "Эскиз1" along normal blind 0.1 contours L4 L5 L6 L7 L8 L9 L10 L11 L12 L13 | L14 A4 L15 A5 L16 A6 L17 A7 L18 A8 L19 A9 L20 A10 L21 A11 L22 A12 L23 A13 L24 A14 L25 A15 L26 A16 L27 A17 L28 A18 L29 A19 | L30 L31 L32 L33 L34 L35 | L36 L37 L38 L39 L40 L41 | L42 L43 L44 L45 L46 L47 | L48 A21 L49 A22 L50 A23 L51 A24 L52 A25 L53 A26 L54 A27 L55 A28 L56 A29 L57 A30 L58 A31 L59 A32 L60 A33 L61 A34 L62 A35 L63 A20 | L64 L65 L66 L67 L68 L69 | L70 L71 L72 L73 L74 L75 | L76 L77 L78 L79 L80 L81 | L82 L83 L84 L85 L86 L87 | L88 A37 L89 A38 L90 A39 L91 A40 L92 A41 L93 A42 L94 A43 L95 A44 L96 A45 L97 A46 L98 A47 L99 A48 L100 A49 L101 A50 L102 A51 L103 A36 | L104 L105 L106 L107 L108 L109 | L110 L111 L112 L113 L114 L115 | L116 A53 L117 A54 L118 A55 L119 A56 L120 A57 L121 A58 L122 A59 L123 A60 L124 A61 L125 A62 L126 A63 L127 A64 L128 A65 L129 A66 L130 A67 L131 A52 | L132 A69 L133 A70 L134 A71 L135 A72 L136 A73 L137 A74 L138 A75 L139 A76 L140 A77 L141 A78 L142 A79 L143 A80 L144 A81 L145 A82 L146 A83 L147 A68 | L148 L149 L150 L151 L152 L153 | L154 A84 L155 A85 L156 A86 L157 A87 L158 A88 L159 A89 L160 A90 L161 A91 L162 A92 L163 A93 L164 A94 L165 A95 L166 A96 L167 A97 L168 A98 L169 A99 | S1 S2 S3 L170 L171 S4 S5 S6 S7 L172 S8 S9 S10 L173 S0 | S12 L174 S13 S14 S15 S16 L175 S17 S18 L176 S19 S20 L177 S21 L178 S22 L179 S23 S24 S25 S26 L180 L181 L182 S27 S28 L183 S11 | L184 S30 S31 L185 S32 S33 L186 S34 S35 L187 S36 S29 | L188 S38 S39 S40 S41 S42 L189 L190 L191 S43 S44 S45 L192 S46 S47 L193 S48 S49 L194 S50 S51 L195 L196 L197 S52 S37 | L198 S54 S55 S56 S57 L199 L200 L201 S58 S59 S60 S61 L202 S62 S63 L203 S64 S65 L204 S66 S67 L205 S68 S53
